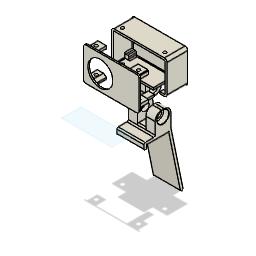
camera_enclosure (Autodesk Fusion 360 design; units mm, degrees)
Autodesk Fusion 360 part; units mm, degrees
sketch "Sketch1" plane through (0, 0, 0) normal (0, 0, 1) x (1, 0, 0)
  line L0 (0, 0) -> (38.5, 0)
  line L1 (38.5, 0) -> (38.5, 21.5)
  line L2 (38.5, 21.5) -> (0, 21.5)
  line L3 (0, 21.5) -> (0, 0)
  dimension "d1" = 38.5
  dimension "d2" = 21.5
  constraint horizontal L0
  constraint vertical L1
  constraint horizontal L2
  constraint vertical L3
  constraint coincident L0.start L3.end
  measures "d1" distance of L0.start L0.end
  measures "d2" distance of L0.start L2.end
extrude "Extrude1" add sketch "Sketch1" along normal blind 2 makes body 1
fillet "Fillet1" radius 2 4 edges at (38.5, 21.5, 1) (0, 21.5, 1) (38.5, 0, 1) (0, 0, 1) on bodies 1
sketch "Sketch2" plane through (0, 0, 2) normal (0, 0, 1) x (1, 0, 0)
  arc A0 (0, 2) -> (2, 0) centre (2, 2) ccw
  line L0 (2, 0) -> (36.5, 0)
  arc A1 (36.5, 0) -> (38.5, 2) centre (36.5, 2) ccw
  line L1 (38.5, 2) -> (38.5, 19.5)
  arc A2 (38.5, 19.5) -> (36.5, 21.5) centre (36.5, 19.5) ccw
  line L2 (36.5, 21.5) -> (2, 21.5)
  arc A3 (2, 21.5) -> (0, 19.5) centre (2, 19.5) ccw
  line L3 (0, 19.5) -> (0, 2)
  circle A4 centre (11, 10) radius 9
  dimension "d7" = 18
  dimension "d8" = 11.5
  dimension "d9" = 11
  measures "d7" diameter of A4
  measures "d8" distance of L2 A4.centre
  measures "d9" distance of L3 A4.centre
extrude "Extrude2" add sketch "Sketch2" along normal blind 20 contours A4 bodies 1
fillet "Fillet2" radius 0.5 1 edges at (2.6091, 6.7455, 22) on bodies 1
sketch "Sketch3" plane through (0, 0, 0) normal (0, 0, -1) x (-1, 0, 0)
  arc A0 (-2, 0) -> (0, 2) centre (-2, 2) ccw
  line L0 (0, 2) -> (0, 19.5)
  arc A1 (0, 19.5) -> (-2, 21.5) centre (-2, 19.5) ccw
  line L1 (-2, 21.5) -> (-36.5, 21.5)
  arc A2 (-36.5, 21.5) -> (-38.5, 19.5) centre (-36.5, 19.5) ccw
  line L2 (-38.5, 19.5) -> (-38.5, 2)
  arc A3 (-38.5, 2) -> (-36.5, 0) centre (-36.5, 2) ccw
  line L3 (-36.5, 0) -> (-2, 0)
  line L4 (-9, 14) -> (-5, 14)
  line L5 (-5, 14) -> (-5, 4)
  line L6 (-5, 4) -> (-9, 4)
  line L7 (-9, 4) -> (-9, 14)
  dimension "d14" = 4
  dimension "d15" = 10
  dimension "d16" = 4
  dimension "d17" = 5
  constraint horizontal L4
  constraint vertical L5
  constraint horizontal L6
  constraint vertical L7
  measures "d14" distance of L5.end L6.end
  measures "d15" distance of L4.start L6.end
  measures "d16" distance of L3 L6
  measures "d17" distance of L0 L5
extrude "Extrude3" add sketch "Sketch3" along normal blind 3 contours L4 L5 L6 L7 bodies 1
fillet "Fillet3" radius 2 2 edges at (9, 9, -3) (5, 9, -3) on bodies 1
sketch "Sketch4" plane through (0, 0, 0) normal (0, 0, -1) x (-1, 0, 0)
  line L0 (-9, 4) -> (-9, 14)
  line L1 (-9, 14) -> (-5, 14)
  line L2 (-5, 14) -> (-5, 4)
  line L3 (-5, 4) -> (-9, 4)
  arc A0 (-2, 0) -> (0, 2) centre (-2, 2) ccw
  line L4 (0, 2) -> (0, 19.5)
  arc A1 (0, 19.5) -> (-2, 21.5) centre (-2, 19.5) ccw
  line L5 (-2, 21.5) -> (-36.5, 21.5)
  arc A2 (-36.5, 21.5) -> (-38.5, 19.5) centre (-36.5, 19.5) ccw
  line L6 (-38.5, 19.5) -> (-38.5, 2)
  arc A3 (-38.5, 2) -> (-36.5, 0) centre (-36.5, 2) ccw
  line L7 (-36.5, 0) -> (-2, 0)
  line L8 (-16, 13) -> (-9, 13)
  line L9 (-9, 13) -> (-9, 6)
  line L10 (-9, 6) -> (-16, 6)
  line L11 (-16, 6) -> (-16, 13)
  dimension "d22" = 7
  dimension "d23" = 7
  dimension "d24" = 6
  constraint horizontal L8
  constraint vertical L9
  constraint horizontal L10
  constraint vertical L11
  constraint collinear L0 L9
  measures "d22" distance of L8.start L8.end
  measures "d23" distance of L8.start L10.end
  measures "d24" distance of L7 L10
extrude "Extrude4" add sketch "Sketch4" along normal blind 1 contours L0 L8 L9 L10 L11 bodies 1
ref_plane "WorkPlane1" through (19.25, 10.75, 10) normal (0, 0, 1) x (1, 0, 0)
sketch "Sketch5" plane through (19.25, 10.75, 10) normal (0, 0, 1) x (1, 0, 0)
  line L0 (19.75, -11.25) -> (-19.75, -11.25)
  line L1 (-19.75, -11.25) -> (-19.75, 11.25)
  line L2 (-19.75, 11.25) -> (19.75, 11.25)
  line L3 (19.75, 11.25) -> (19.75, -11.25)
  line L4 (19.25, -8.75) -> (19.25, 8.75)
  line L5 (-19.25, 8.75) -> (-19.25, -8.75)
  line L6 (17.25, 10.75) -> (-17.25, 10.75)
  line L7 (-17.25, -10.75) -> (17.25, -10.75)
  line L8 (-21.25, -12.75) -> (-21.25, 12.75)
  line L9 (-21.25, 12.75) -> (21.25, 12.75)
  line L10 (21.25, 12.75) -> (21.25, -12.75)
  line L11 (21.25, -12.75) -> (-21.25, -12.75)
  circle A0 centre (-8.25, -0.75) radius 8.5
  circle A1 centre (-8.25, -0.75) radius 9.5
  dimension "d28" = 0.5
  dimension "d29" = 0.5
  dimension "d30" = 0.5
  dimension "d31" = 0.5
  dimension "d32" = -1.5
  dimension "d33" = 19
  constraint horizontal L0
  constraint vertical L1
  constraint horizontal L2
  constraint vertical L3
  constraint concentric A0 A1
  measures "d28" distance of L3 L4
  measures "d29" distance of L1 L5
  measures "d30" distance of L2 L6
  measures "d31" distance of L0 L7
  measures "d33" diameter of A1
extrude "Extrude5" add sketch "Sketch5" along normal blind 1.2 separate body contours L0 L1 L2 L3 | L8 L9 L10 L11 makes body 2
fillet "Fillet4" radius 2 4 edges at (40.5, 23.5, 10.6) (-2, 23.5, 10.6) (-2, -2, 10.6) (40.5, -2, 10.6) on bodies 2
sketch "Sketch6" plane through (0, 0, 10) normal (0, 0, -1) x (-1, 0, 0)
  circle A0 centre (-11, 10) radius 9.5
  arc A1 (-40.5, 0) -> (-38.5, -2) centre (-38.5, 0) ccw
  line L0 (-38.5, -2) -> (0, -2)
  arc A2 (0, -2) -> (2, 0) centre (0, 0) ccw
  line L1 (2, 0) -> (2, 21.5)
  arc A3 (2, 21.5) -> (0, 23.5) centre (0, 21.5) ccw
  line L2 (0, 23.5) -> (-38.5, 23.5)
  arc A4 (-38.5, 23.5) -> (-40.5, 21.5) centre (-38.5, 21.5) ccw
  line L3 (-40.5, 21.5) -> (-40.5, 0)
  line L4 (-39, 21.5) -> (-39, 0)
  arc A5 (-39, 0) -> (-38.5, -0.5) centre (-38.5, 0) ccw
  line L5 (-38.5, -0.5) -> (0, -0.5)
  arc A6 (0, -0.5) -> (0.5, 0) centre (0, 0) ccw
  line L6 (0.5, 0) -> (0.5, 21.5)
  arc A7 (0.5, 21.5) -> (0, 22) centre (0, 21.5) ccw
  line L7 (0, 22) -> (-38.5, 22)
  arc A8 (-38.5, 22) -> (-39, 21.5) centre (-38.5, 21.5) ccw
  dimension "d38" = -1.5
extrude "Extrude6" add sketch "Sketch6" along normal blind 15 separate body contours A1 L0 A2 L1 A3 L2 A4 L3 makes body 3
sketch "Sketch7" plane through (0, 0, -5) normal (0, 0, -1) x (-1, 0, 0)
  arc A0 (-38.5, 22) -> (-39, 21.5) centre (-38.5, 21.5) ccw
  line L0 (-38.5, 22) -> (0, 22)
  arc A1 (0.5, 21.5) -> (0, 22) centre (0, 21.5) ccw
  line L1 (0.5, 21.5) -> (0.5, 0)
  arc A2 (0, -0.5) -> (0.5, 0) centre (0, 0) ccw
  line L2 (0, -0.5) -> (-38.5, -0.5)
  arc A3 (-39, 0) -> (-38.5, -0.5) centre (-38.5, 0) ccw
  line L3 (-39, 0) -> (-39, 21.5)
  line L4 (-40.5, 21.5) -> (-40.5, 0)
  arc A4 (-40.5, 0) -> (-38.5, -2) centre (-38.5, 0) ccw
  line L5 (-38.5, -2) -> (0, -2)
  arc A5 (0, -2) -> (2, 0) centre (0, 0) ccw
  line L6 (2, 0) -> (2, 21.5)
  arc A6 (2, 21.5) -> (0, 23.5) centre (0, 21.5) ccw
  line L7 (0, 23.5) -> (-38.5, 23.5)
  arc A7 (-38.5, 23.5) -> (-40.5, 21.5) centre (-38.5, 21.5) ccw
extrude "Extrude7" add sketch "Sketch7" along normal blind 1.2 contours A0 L0 A1 L1 A2 L2 A3 L3 | L4 A4 L5 A5 L6 A6 L7 A7 bodies 3
sketch "Sketch8" plane through (0, 0, -6.2) normal (0, 0, -1) x (-1, 0, 0)
  arc A0 (-38.5, 23.5) -> (-40.5, 21.5) centre (-38.5, 21.5) ccw
  line L0 (-40.5, 21.5) -> (-40.5, 0)
  arc A1 (-40.5, 0) -> (-38.5, -2) centre (-38.5, 0) ccw
  line L1 (-38.5, -2) -> (0, -2)
  arc A2 (0, -2) -> (2, 0) centre (0, 0) ccw
  line L2 (2, 0) -> (2, 21.5)
  arc A3 (2, 21.5) -> (0, 23.5) centre (0, 21.5) ccw
  line L3 (0, 23.5) -> (-38.5, 23.5)
  circle A4 centre (-32.5, 2.5) radius 2.5
  arc A5 (-38.5, 22) -> (-39, 21.5) centre (-38.5, 21.5) ccw
  line L4 (-39, 21.5) -> (-39, 0)
  arc A6 (-39, 0) -> (-38.5, -0.5) centre (-38.5, 0) ccw
  line L5 (-38.5, -0.5) -> (0, -0.5)
  arc A7 (0, -0.5) -> (0.5, 0) centre (0, 0) ccw
  line L6 (0.5, 0) -> (0.5, 21.5)
  arc A8 (0.5, 21.5) -> (0, 22) centre (0, 21.5) ccw
  line L7 (0, 22) -> (-38.5, 22)
  line L8 (-40.5, 0) -> (-40.5, 21.5)
  arc A9 (-38.5, 23.5) -> (-40.5, 21.5) centre (-38.5, 21.5) ccw
  line L9 (-38.5, 23.5) -> (0, 23.5)
  arc A10 (2, 21.5) -> (0, 23.5) centre (0, 21.5) ccw
  line L10 (2, 21.5) -> (2, 0)
  arc A11 (0, -2) -> (2, 0) centre (0, 0) ccw
  line L11 (0, -2) -> (-38.5, -2)
  arc A12 (-40.5, 0) -> (-38.5, -2) centre (-38.5, 0) ccw
  line L12 (-32.5, 2.5) -> (-30, 2.5) construction
  line L13 (-32.5, 2.5) -> (-35, 2.5) construction
  line L14 (-30, 2.5) -> (-30, -0.5)
  line L15 (-35, 2.5) -> (-35, -0.5)
  dimension "d43" = 5
  dimension "d44" = 4.5
  dimension "d45" = 8
  constraint coincident A4.centre L12.start
  constraint coincident A4 L12.end
  constraint horizontal L12
  constraint coincident A4 L13.end
  constraint parallel L12 L13
  constraint coincident L5 L14.end
  constraint tangent A4 L14
  constraint coincident L5 L15.end
  constraint tangent A4 L15
  measures "d43" diameter of A4
  measures "d44" distance of L1 A4.centre
  measures "d45" distance of L0 A4.centre
extrude "Extrude22" cut sketch "Sketch8" against normal blind 1.2 contours A4 L5 L14 L15 bodies 3
extrude "Extrude8" cut sketch "Sketch8" against normal blind 1.2 contours A4 bodies 3
sketch "Sketch21" plane through (0, -0.5, 0) normal (0, 1, 0) x (-1, 0, 0)
  line L0 (0, 10) -> (-38.5, 10)
  line L1 (-38.5, 10) -> (-38.5, -5)
  line L2 (-38.5, -5) -> (-35, -5)
  line L3 (-35, -5) -> (-35, -6.2)
  line L4 (-35, -6.2) -> (-30, -6.2)
  line L5 (-30, -6.2) -> (-30, -5)
  line L6 (-30, -5) -> (0, -5)
  line L7 (0, -5) -> (0, 10)
sketch "Sketch22" plane through (0, -2, 0) normal (0, -1, 0) x (1, 0, 0)
  line L0 (38.5, 10) -> (0, 10)
  line L1 (0, 10) -> (0, -6.2)
  line L2 (0, -6.2) -> (38.5, -6.2)
  line L3 (38.5, -6.2) -> (38.5, 10)
  line L4 (30, -6.2) -> (30, -5)
  line L5 (30, -5) -> (30, -6.2)
  line L6 (35, -6.2) -> (35, -5)
  line L7 (35, -5) -> (35, -6.2)
  line L8 (35, -6.2) -> (30, -6.2)
  line L9 (30, -5) -> (30, 10)
  line L10 (35, -5) -> (35, 10)
  line L11 (30, 10) -> (35, 10)
  constraint coincident L6.start L7.end
  constraint coincident L4.start L5.end
  constraint coincident L4.end L5.start
  constraint coincident L0 L9.end
  constraint perpendicular L0 L9
  constraint coincident L6.end L7.start
  constraint coincident L0 L10.end
  constraint perpendicular L0 L10
extrude "Extrude23" cut sketch "Sketch22" against normal blind 1.5 contours L0 L2 L4 L5 L6 L7 L8 L9 L10 L11 bodies 3
chamfer "Chamfer1" distance 0.5 angle 45 8 edges at (19.25, 22, -5) (-0.3536, 21.8536, -5) (-0.5, 10.75, -5) (-0.3536, -0.3536, -5) (19.25, -0.5, -5) (38.8536, -0.3536, -5) (39, 10.75, -5) (38.8536, 21.8536, -5) on bodies 3
fillet "Fillet5" radius 0.3 8 edges at (40.5, 10.75, -6.2) (39.9142, -1.4142, -6.2) (19.25, -2, -6.2) (-1.4142, -1.4142, -6.2) (-2, 10.75, -6.2) (-1.4142, 22.9142, -6.2) (19.25, 23.5, -6.2) (39.9142, 22.9142, -6.2) on bodies 3
sketch "Sketch10" plane through (0, 0, 22) normal (0, 0, 1) x (1, 0, 0)
  circle A0 centre (11, 10) radius 8.5
  circle A1 centre (11, 10) radius 6.0027
  constraint concentric A0 A1
extrude "Extrude10" cut sketch "Sketch10" against normal blind 5 contours A1 bodies 1
chamfer "Chamfer3" distance 2 angle 45 2 edges at (5.4035, 12.1707, 22) (5.4035, 12.1707, 17) on bodies 1
move_body "Move1" bodies 3 to x (1, 0, 0) y (0, 1, 0) z (0, 0, 1) at (0, 0, -40)
move_body "Move2" bodies 1 to x (1, 0, 0) y (0, 1, 0) z (0, 0, 1) at (0, 0, -20)
ref_plane "WorkPlane2" through (19.25, 10.75, -37.95) normal (1, 0, 0) x (0, -1, 0)
sketch "Sketch11" plane through (19.25, 10.75, -37.95) normal (1, 0, 0) x (0, 0, -1)
  line L0 (7.95, -12.75) -> (7.95, -10.75)
  line L1 (7.95, -10.75) -> (-7.95, -10.75)
  line L2 (-7.95, -12.75) -> (-7.95, -10.75)
  line L3 (-7.95, -12.75) -> (7.95, -12.75)
  line L4 (-5.85, -12.75) -> (6.15, -12.75)
  line L5 (6.15, -12.75) -> (6.15, -24.75)
  line L6 (6.15, -24.75) -> (-5.85, -24.75)
  line L7 (-5.85, -24.75) -> (-5.85, -12.75)
  line L8 (8.25, -10.75) -> (8.25, 10.75)
  dimension "d71" = 2.1
  dimension "d73" = 12
  dimension "d74" = 2.2
  dimension "d75" = 12
  constraint horizontal L4
  constraint vertical L5
  constraint horizontal L6
  constraint vertical L7
  constraint coincident L3 L4.start
  measures "d71" distance of L5 L8
  measures "d73" distance of L5 L7
  measures "d75" distance of L4.start L6.end
extrude "Extrude11" add sketch "Sketch11" along normal mid plane 6 contours L3 L4 L5 L6 L7 bodies 3
ref_plane "WorkPlane3" through (22.55, -8, -38.1) normal (1, 0, 0) x (0, 0, -1)
sketch "Sketch12" plane through (22.55, -8, -38.1) normal (1, 0, 0) x (0, 0, -1)
  line L0 (-6, -6) -> (6, -6)
  line L1 (6, -6) -> (6, 6)
  line L2 (6, 6) -> (-6, 6)
  line L3 (-6, 6) -> (-6, -6)
  line L4 (6, 4) -> (-6, 4)
  line L5 (-6, -6) -> (6, -6)
  line L6 (6, -6) -> (6, -11)
  line L7 (6, -11) -> (-6, -11)
  line L8 (-6, -11) -> (-6, -6)
  dimension "d79" = 2
  dimension "d80" = 5
  constraint coincident L1 L4.start
  constraint coincident L3 L4.end
  constraint perpendicular L3 L4
  constraint horizontal L5
  constraint vertical L6
  constraint horizontal L7
  constraint vertical L8
  constraint coincident L0.start L3.end
  constraint collinear L1 L6
  measures "d79" distance of L2 L4
  measures "d80" distance of L0.end L6.end
extrude "Extrude12" add sketch "Sketch12" along normal blind 3 separate body contours L0 L1 L3 L4 L5 | L0 L5 L6 L7 L8 makes body 4
ref_plane "WorkPlane4" through (19.25, -8, -38.1) normal (-1, 0, 0) x (0, 0, 1)
mirror "Mirror1" about plane through (19.25, -8, -38.1) normal (-1, 0, 0) of bodies 4 makes body 5
sketch "Sketch13" plane through (0, -19, 0) normal (0, -1, 0) x (1, 0, 0)
  line L0 (22.55, -32.1) -> (22.55, -44.1)
  line L1 (22.55, -44.1) -> (25.55, -44.1)
  line L2 (25.55, -44.1) -> (25.55, -32.1)
  line L3 (25.55, -32.1) -> (22.55, -32.1)
  line L4 (15.95, -44.1) -> (15.95, -32.1)
  line L5 (15.95, -32.1) -> (12.95, -32.1)
  line L6 (12.95, -32.1) -> (12.95, -44.1)
  line L7 (12.95, -44.1) -> (15.95, -44.1)
  line L8 (15.95, -32.1) -> (22.55, -32.1)
  line L9 (22.55, -32.1) -> (22.55, -44.1)
  line L10 (22.55, -44.1) -> (15.95, -44.1)
  line L11 (15.95, -44.1) -> (15.95, -32.1)
  constraint horizontal L8
  constraint vertical L9
  constraint horizontal L10
  constraint vertical L11
  constraint coincident L0.end L1.start
  constraint coincident L4.end L5.start
extrude "Extrude13" add sketch "Sketch13" against normal blind 2 contours L0 L4 L8 L9 L10 L11 bodies 4 5
fillet "Fillet7" radius 5 6 edges at (19.25, -14, -32.1) (19.25, -14, -44.1) (24.05, -4, -44.1) (24.05, -4, -32.1) (14.45, -4, -32.1) (14.45, -4, -44.1) on bodies 3 4
sketch "Sketch14" plane through (12.95, 0, 0) normal (-1, 0, 0) x (0, 0, 1)
  arc A0 (-39.1, -4) -> (-44.1, -9) centre (-39.1, -9) ccw
  line L0 (-44.1, -9) -> (-44.1, -19)
  line L1 (-44.1, -19) -> (-32.1, -19)
  line L2 (-32.1, -19) -> (-32.1, -9)
  arc A1 (-32.1, -9) -> (-37.1, -4) centre (-37.1, -9) ccw
  line L3 (-37.1, -4) -> (-39.1, -4)
  circle A2 centre (-38.1, -9) radius 3
  dimension "d90" = 6
  dimension "d91" = 6
  dimension "d92" = 6
  dimension "d93" = 5
  measures "d90" distance of L2 A2.centre
  measures "d91" distance of L0 A2.centre
  measures "d92" diameter of A2
  measures "d93" distance of L3 A2.centre
extrude "Extrude14" cut sketch "Sketch14" against normal blind 13 contours A2 bodies 3 4
sketch "Sketch15" plane through (12.95, 0, 0) normal (-1, 0, 0) x (0, 0, 1)
  circle A0 centre (-38.1, -9) radius 3
  arc A1 (-39.1, -4) -> (-44.1, -9) centre (-39.1, -9) ccw
  line L0 (-44.1, -9) -> (-44.1, -19)
  line L1 (-44.1, -19) -> (-32.1, -19)
  line L2 (-32.1, -19) -> (-32.1, -9)
  arc A2 (-32.1, -9) -> (-37.1, -4) centre (-37.1, -9) ccw
  line L3 (-37.1, -4) -> (-39.1, -4)
  line L4 (-35.6751, -4.8) -> (-40.5249, -4.8)
  line L5 (-40.5249, -4.8) -> (-42.9497, -9)
  line L6 (-42.9497, -9) -> (-40.5249, -13.2)
  line L7 (-40.5249, -13.2) -> (-35.6751, -13.2)
  line L8 (-35.6751, -13.2) -> (-33.2503, -9)
  line L9 (-33.2503, -9) -> (-35.6751, -4.8)
  line L10 (-42.9497, -9) -> (-33.2503, -9) construction
  point P0 (-38.1, -9)
  dimension "d96" = 4.2
  constraint coincident P0 A0.centre
  constraint parallel L1 L7
  measures "d96" distance of P0 L9
extrude "Extrude15" add sketch "Sketch15" along normal blind 4 contours A1 L0 L1 L2 A2 L3 bodies 4
sketch "Sketch16" plane through (25.55, 0, 0) normal (1, 0, 0) x (0, 0, -1)
  circle A0 centre (38.1, -9) radius 3
  arc A1 (37.1, -4) -> (32.1, -9) centre (37.1, -9) ccw
  line L0 (32.1, -9) -> (32.1, -19)
  line L1 (32.1, -19) -> (44.1, -19)
  line L2 (44.1, -19) -> (44.1, -9)
  arc A2 (44.1, -9) -> (39.1, -4) centre (39.1, -9) ccw
  line L3 (39.1, -4) -> (37.1, -4)
  circle A3 centre (38.1, -9) radius 4.5
  dimension "d99" = 9
  constraint concentric A0 A3
  measures "d99" diameter of A3
extrude "Extrude16" add sketch "Sketch16" along normal blind 4 contours A1 L0 L1 L2 A2 L3 bodies 4
chamfer "Chamfer4" distance 0.2 angle 45 6 edges at (8.95, -4.8, -38.1) (8.95, -6.9, -41.7373) (8.95, -11.1, -41.7373) (8.95, -6.9, -34.4627) (8.95, -11.1, -34.4627) (8.95, -13.2, -38.1) on bodies 4
chamfer "Chamfer5" distance 0.2 angle 45 1 edges at (29.55, -7.3727, -33.9045) on bodies 4
move_body "Move3" bodies 3 1 2 to x (1, 0, 0) y (0, 1, 0) z (0, 0, 1) at (0, 15, 0)
sketch "Sketch17" plane through (29.55, 0, 0) normal (1, 0, 0) x (0, 0, -1)
  line L0 (39.1, -4) -> (37.1, -4)
  arc A0 (37.1, -4) -> (32.1, -9) centre (37.1, -9) ccw
  line L1 (32.1, -9) -> (32.1, -19)
  line L2 (32.1, -19) -> (44.1, -19)
  line L3 (44.1, -19) -> (44.1, -9)
  arc A1 (44.1, -9) -> (39.1, -4) centre (39.1, -9) ccw
  circle A2 centre (38.1, -9) radius 4.7
  line L4 (32.1, -19) -> (23.4688, -19)
  line L5 (23.4688, -19) -> (23.4688, -24)
  line L6 (23.4688, -24) -> (25.4688, -24)
  line L7 (25.4688, -24) -> (25.4688, -21)
  line L8 (25.4688, -21) -> (42.4688, -21)
  line L9 (42.4688, -21) -> (51.5173, -65.0809)
  line L10 (51.5173, -65.0809) -> (53.4765, -64.6787)
  line L11 (53.4765, -64.6787) -> (44.1, -19)
  dimension "d104" = 2
  dimension "d105" = 17
  dimension "d107" = 2
  dimension "d108" = 2
  dimension "d109" = 45
  dimension "d110" = 11.6
  dimension "d111" = 5
  constraint coincident L1.end L2.start
  constraint perpendicular L1 L4
  constraint perpendicular L4 L5
  constraint perpendicular L5 L6
  constraint perpendicular L6 L7
  constraint perpendicular L7 L8
  constraint perpendicular L9 L10
  constraint perpendicular L10 L11
  constraint coincident L2.end L3.start
  measures "d104" distance of L9 L11
  measures "d105" distance of L7 L8.end
  measures "d107" distance of L5 L7
  measures "d108" distance of L2 L8
  measures "d109" distance of L8.end L9.end
  measures "d110" angle of L7 L9
  measures "d111" distance of L4 L6
extrude "Extrude18" add sketch "Sketch17" against normal blind 20.6 contours L2 L4 L5 L6 L7 L8 L9 L10 L11 bodies 4
extrude "Extrude17" add sketch "Sketch17" against normal blind 20.6 contours L2 L4 L5 L6 L7 L8 L9 L10 L11 bodies 4
fillet "Fillet8" radius 10 1 edges at (19.25, -19, -44.1) on bodies 4
sketch "Sketch18" plane through (8.95, 0, 0) normal (-1, 0, 0) x (0, 0, 1)
  line L0 (-35.5597, -13.4) -> (-40.6403, -13.4)
  line L1 (-40.6403, -13.4) -> (-43.1807, -9)
  line L2 (-43.1807, -9) -> (-40.6403, -4.6)
  line L3 (-40.6403, -4.6) -> (-35.5597, -4.6)
  line L4 (-35.5597, -4.6) -> (-33.0193, -9)
  line L5 (-33.0193, -9) -> (-35.5597, -13.4)
  line L6 (-32.1, -19) -> (-32.1, -9)
  arc A0 (-32.1, -9) -> (-37.1, -4) centre (-37.1, -9) ccw
  line L7 (-37.1, -4) -> (-39.1, -4)
  arc A1 (-39.1, -4) -> (-44.1, -9) centre (-39.1, -9) ccw
  line L8 (-44.1, -9) -> (-44.1, -17.9842)
  arc A2 (-44.3042, -19.995) -> (-44.1, -17.9842) centre (-54.1, -17.9842) ccw
  line L9 (-44.3042, -19.995) -> (-53.4765, -64.6787)
  line L10 (-53.4765, -64.6787) -> (-51.5173, -65.0809)
  line L11 (-51.5173, -65.0809) -> (-42.4688, -21)
  line L12 (-42.4688, -21) -> (-25.4688, -21)
  line L13 (-25.4688, -21) -> (-25.4688, -24)
  line L14 (-25.4688, -24) -> (-23.4688, -24)
  line L15 (-23.4688, -24) -> (-23.4688, -19)
  line L16 (-23.4688, -19) -> (-32.1, -19)
  circle A3 centre (-42.4688, -21) radius 0.4
  circle A4 centre (-25.4688, -21) radius 0.4
  dimension "d118" = 0.8
  dimension "d119" = 0.8
  constraint coincident L11.end L12.start
  constraint coincident L12.end L13.start
  measures "d118" diameter of A3
  measures "d119" diameter of A4
extrude "Extrude19" cut sketch "Sketch18" against normal blind 20.6 contours L12 L13 A4 | L11 L12 A3 picked at (-25.4688, -20.7341) picked at (-42.693, -21.1431) bodies 4
fillet "Fillet9" radius 1 8 edges at (19.25, -24, -25.4688) (19.25, -24, -23.4688) (19.25, -19, -23.4688) (19.25, -19, -32.1) (19.25, -65.0809, -51.5173) (19.25, -64.6787, -53.4765) (19.25, -17, -44.1) (19.25, -17, -32.1) on bodies 4
sketch "Sketch20" plane through (0, 0, -45) normal (0, 0, 1) x (1, 0, 0)
  line L0 (38.5, 36.5) -> (0, 36.5)
  line L1 (0, 36.5) -> (0, 15)
  line L2 (35, 15) -> (38.5, 15)
  line L3 (38.5, 15) -> (38.5, 36.5)
  arc A0 (39, 36.5) -> (38.5, 37) centre (38.5, 36.5) ccw
  line L4 (39, 36.5) -> (39, 15)
  arc A1 (38.5, 14.5) -> (39, 15) centre (38.5, 15) ccw
  line L5 (30, 14.5) -> (0, 14.5)
  arc A2 (-0.5, 15) -> (0, 14.5) centre (0, 15) ccw
  line L6 (-0.5, 15) -> (-0.5, 36.5)
  arc A3 (0, 37) -> (-0.5, 36.5) centre (0, 36.5) ccw
  line L7 (0, 37) -> (38.5, 37)
  line L8 (40.5, 15) -> (40.5, 36.5)
  arc A4 (40.5, 36.5) -> (38.5, 38.5) centre (38.5, 36.5) ccw
  line L9 (38.5, 38.5) -> (0, 38.5)
  arc A5 (0, 38.5) -> (-2, 36.5) centre (0, 36.5) ccw
  line L10 (-2, 36.5) -> (-2, 15)
  arc A6 (-2, 15) -> (0, 13) centre (0, 15) ccw
  line L11 (35, 13) -> (38.5, 13)
  arc A7 (38.5, 13) -> (40.5, 15) centre (38.5, 15) ccw
  line L12 (2.5, 37) -> (2.5, 34)
  line L13 (2.5, 34) -> (-0.5, 34)
  line L14 (36, 37) -> (36, 34)
  line L15 (36, 34) -> (39, 34)
  line L16 (36, 14.5) -> (36, 17.5)
  line L17 (36, 17.5) -> (39, 17.5)
  line L18 (-0.5, 17.5) -> (2.5, 17.5)
  line L19 (2.5, 17.5) -> (2.5, 14.5)
  line L20 (0, 15) -> (30, 15)
  line L21 (30, 15) -> (30, 17.5)
  arc A8 (35, 17.5) -> (30, 17.5) centre (32.5, 17.5) ccw
  line L22 (35, 17.5) -> (35, 15)
  line L23 (30, 13) -> (30, 14.5)
  line L24 (38.5, 14.5) -> (35, 14.5)
  line L25 (35, 14.5) -> (35, 13)
  line L26 (0, 13) -> (30, 13)
  dimension "d130" = 3
  dimension "d131" = 3
  dimension "d132" = 3
  dimension "d133" = 3
  dimension "d134" = 3
  dimension "d135" = 3
  dimension "d136" = 3
  dimension "d137" = 3
  constraint coincident L7 L12.start
  constraint perpendicular L0 L12
  constraint coincident L6 L13.end
  constraint perpendicular L6 L13
  constraint coincident L7 L14.start
  constraint perpendicular L0 L14
  constraint coincident L4 L15.end
  constraint perpendicular L4 L15
  constraint coincident L5 L16.start
  constraint perpendicular L2 L16
  constraint coincident L4 L17.end
  constraint perpendicular L4 L17
  constraint coincident L6 L18.start
  constraint perpendicular L1 L18
  constraint coincident L5 L19.end
  constraint perpendicular L5 L19
  measures "d130" distance of L12.start L12.end
  measures "d131" distance of L12.end L13.end
  measures "d132" distance of L18.end L19.end
  measures "d133" distance of L18.start L18.end
  measures "d134" distance of L14.start L14.end
  measures "d135" distance of L14.end L15.end
  measures "d136" distance of L16.end L17.end
  measures "d137" distance of L16.start L16.end
extrude "Extrude21" add sketch "Sketch20" along normal blind 6 contours L0 L3 L14 L15 | L0 L3 A0 L4 L7 L14 L15 | L0 L1 L12 L13 | L0 L1 L6 A3 L7 L12 L13 | L2 L3 L4 A1 L16 L17 L24 | L2 L3 L16 L17 | L1 L18 L19 L20 | L1 L5 A2 L6 L18 L19 L20 bodies 3
fillet "Fillet10" radius 0.8 12 edges at (39, 34, -41.75) (36, 37, -41.75) (36, 34, -42) (39, 17.5, -41.75) (36, 17.5, -42) (36, 14.5, -41.75) (2.5, 37, -41.75) (2.5, 34, -42) (-0.5, 34, -41.75) (-0.5, 17.5, -41.75) (2.5, 17.5, -42) (2.5, 14.5, -41.75) on bodies 3
move_body "Move4" bodies 2 to x (1, 0, 0) y (0, 1, 0) z (0, 0, 1) at (0, 0, -40)
sketch "Sketch23" plane through (0, 0, -30) normal (0, 0, -1) x (-1, 0, 0)
  circle A0 centre (-11, 25) radius 9.5
  arc A1 (-40.5, 15) -> (-38.5, 13) centre (-38.5, 15) ccw
  line L0 (-38.5, 13) -> (0, 13)
  arc A2 (0, 13) -> (2, 15) centre (0, 15) ccw
  line L1 (2, 15) -> (2, 36.5)
  arc A3 (2, 36.5) -> (0, 38.5) centre (0, 36.5) ccw
  line L2 (0, 38.5) -> (-38.5, 38.5)
  arc A4 (-38.5, 38.5) -> (-40.5, 36.5) centre (-38.5, 36.5) ccw
  line L3 (-40.5, 36.5) -> (-40.5, 15)
  arc A5 (-2.5, 34.8) -> (-1.7, 34) centre (-1.7, 34.8) ccw
  line L4 (-2.5, 34.8) -> (-2.5, 36.2)
  arc A6 (-2.5, 36.2) -> (-3.3, 37) centre (-3.3, 36.2) ccw
  line L5 (-3.3, 37) -> (0, 37)
  arc A7 (0.5, 36.5) -> (0, 37) centre (0, 36.5) ccw
  line L6 (0.5, 36.5) -> (0.5, 33.2)
  arc A8 (0.5, 33.2) -> (-0.3, 34) centre (-0.3, 33.2) ccw
  line L7 (-0.3, 34) -> (-1.7, 34)
  arc A9 (-1.7, 17.5) -> (-2.5, 16.7) centre (-1.7, 16.7) ccw
  line L8 (-1.7, 17.5) -> (-0.3, 17.5)
  arc A10 (-0.3, 17.5) -> (0.5, 18.3) centre (-0.3, 18.3) ccw
  line L9 (0.5, 18.3) -> (0.5, 15)
  arc A11 (0, 14.5) -> (0.5, 15) centre (0, 15) ccw
  line L10 (0, 14.5) -> (-3.3, 14.5)
  arc A12 (-3.3, 14.5) -> (-2.5, 15.3) centre (-3.3, 15.3) ccw
  line L11 (-2.5, 15.3) -> (-2.5, 16.7)
  arc A13 (-36, 16.7) -> (-36.8, 17.5) centre (-36.8, 16.7) ccw
  line L12 (-36, 16.7) -> (-36, 15.3)
  arc A14 (-36, 15.3) -> (-35.2, 14.5) centre (-35.2, 15.3) ccw
  line L13 (-35.2, 14.5) -> (-38.5, 14.5)
  arc A15 (-39, 15) -> (-38.5, 14.5) centre (-38.5, 15) ccw
  line L14 (-39, 15) -> (-39, 18.3)
  arc A16 (-39, 18.3) -> (-38.2, 17.5) centre (-38.2, 18.3) ccw
  line L15 (-38.2, 17.5) -> (-36.8, 17.5)
  arc A17 (-36.8, 34) -> (-36, 34.8) centre (-36.8, 34.8) ccw
  line L16 (-36.8, 34) -> (-38.2, 34)
  arc A18 (-38.2, 34) -> (-39, 33.2) centre (-38.2, 33.2) ccw
  line L17 (-39, 33.2) -> (-39, 36.5)
  arc A19 (-38.5, 37) -> (-39, 36.5) centre (-38.5, 36.5) ccw
  line L18 (-38.5, 37) -> (-35.2, 37)
  arc A20 (-35.2, 37) -> (-36, 36.2) centre (-35.2, 36.2) ccw
  line L19 (-36, 36.2) -> (-36, 34.8)
extrude "Extrude24" add sketch "Sketch23" along normal up to surface (7.8 mm away) contours A5 L4 A6 L5 A7 L6 A8 L7 | A9 L8 A10 L9 A11 L10 A12 L11 | A13 L12 A14 L13 A15 L14 A16 L15 | A17 L16 A18 L17 A19 L18 A20 L19 bodies 2
sketch "Sketch24" plane through (0, 0, -37.8) normal (0, 0, -1) x (-1, 0, 0)
  line L0 (-35.2, 37) -> (-38.5, 37)
  arc A0 (-38.5, 37) -> (-39, 36.5) centre (-38.5, 36.5) ccw
  line L1 (-39, 36.5) -> (-39, 33.2)
  arc A1 (-38.2, 34) -> (-39, 33.2) centre (-38.2, 33.2) ccw
  line L2 (-38.2, 34) -> (-36.8, 34)
  arc A2 (-36.8, 34) -> (-36, 34.8) centre (-36.8, 34.8) ccw
  line L3 (-36, 34.8) -> (-36, 36.2)
  arc A3 (-35.2, 37) -> (-36, 36.2) centre (-35.2, 36.2) ccw
  line L4 (-38.2, 34) -> (-39, 34)
  line L5 (-36, 36.2) -> (-36, 37)
  line L6 (0.5, 33.2) -> (0.5, 36.5)
  arc A4 (0.5, 36.5) -> (0, 37) centre (0, 36.5) ccw
  line L7 (0, 37) -> (-3.3, 37)
  arc A5 (-2.5, 36.2) -> (-3.3, 37) centre (-3.3, 36.2) ccw
  line L8 (-2.5, 36.2) -> (-2.5, 34.8)
  arc A6 (-2.5, 34.8) -> (-1.7, 34) centre (-1.7, 34.8) ccw
  line L9 (-1.7, 34) -> (-0.3, 34)
  arc A7 (0.5, 33.2) -> (-0.3, 34) centre (-0.3, 33.2) ccw
  line L10 (-3.3, 14.5) -> (0, 14.5)
  arc A8 (0, 14.5) -> (0.5, 15) centre (0, 15) ccw
  line L11 (0.5, 15) -> (0.5, 18.3)
  arc A9 (-0.3, 17.5) -> (0.5, 18.3) centre (-0.3, 18.3) ccw
  line L12 (-0.3, 17.5) -> (-1.7, 17.5)
  arc A10 (-1.7, 17.5) -> (-2.5, 16.7) centre (-1.7, 16.7) ccw
  line L13 (-2.5, 16.7) -> (-2.5, 15.3)
  arc A11 (-3.3, 14.5) -> (-2.5, 15.3) centre (-3.3, 15.3) ccw
  line L14 (-39, 18.3) -> (-39, 15)
  arc A12 (-39, 15) -> (-38.5, 14.5) centre (-38.5, 15) ccw
  line L15 (-38.5, 14.5) -> (-35.2, 14.5)
  arc A13 (-36, 15.3) -> (-35.2, 14.5) centre (-35.2, 15.3) ccw
  line L16 (-36, 15.3) -> (-36, 16.7)
  arc A14 (-36, 16.7) -> (-36.8, 17.5) centre (-36.8, 16.7) ccw
  line L17 (-36.8, 17.5) -> (-38.2, 17.5)
  arc A15 (-39, 18.3) -> (-38.2, 17.5) centre (-38.2, 18.3) ccw
  line L18 (-0.3, 34) -> (0.5, 34)
  line L19 (-2.5, 36.2) -> (-2.5, 37)
  line L20 (-0.3, 17.5) -> (0.5, 17.5)
  line L21 (-2.5, 15.3) -> (-2.5, 14.5)
  line L22 (-36, 15.3) -> (-36, 14.5)
  line L23 (-38.2, 17.5) -> (-39, 17.5)
  line L24 (-38.8, 34) -> (-38.8, 36.9)
  line L25 (-36, 36.8) -> (-38.9, 36.8)
  line L26 (-2.5, 36.8) -> (0.4, 36.8)
  line L27 (0.3, 34) -> (0.3, 36.9)
  line L28 (0.3, 17.5) -> (0.3, 14.6)
  line L29 (-2.5, 14.7) -> (0.4, 14.7)
  line L30 (-36, 14.7) -> (-38.9, 14.7)
  line L31 (-38.8, 17.5) -> (-38.8, 14.6)
  dimension "d149" = 0.2
  dimension "d150" = 0.2
  dimension "d151" = 0.2
  dimension "d152" = 0.2
  dimension "d153" = 0.2
  dimension "d154" = 0.2
  dimension "d155" = 0.2
  dimension "d156" = 0.2
  constraint coincident A1.start L2.start
  constraint coincident L1 L4.end
  constraint tangent A1 L4
  constraint coincident L3.end A3.end
  constraint coincident L0 L5.end
  constraint tangent A3 L5
  constraint coincident L9.end A7.end
  constraint coincident L6 L18.end
  constraint tangent A7 L18
  constraint coincident A5.start L8.start
  constraint coincident L7 L19.end
  constraint tangent A5 L19
  constraint coincident A9.start L12.start
  constraint coincident L11 L20.end
  constraint tangent A9 L20
  constraint coincident L13.end A11.end
  constraint coincident L10 L21.end
  constraint tangent A11 L21
  constraint coincident A13.start L16.start
  constraint coincident L15 L22.end
  constraint tangent A13 L22
  constraint coincident L17.end A15.end
  constraint coincident L14 L23.end
  constraint tangent A15 L23
  constraint coincident L4 L24.start
  constraint perpendicular L0 L24
  constraint coincident A0 L24.end
  constraint coincident L5 L25.start
  constraint coincident A0 L25.end
  constraint perpendicular L24 L25
  constraint coincident L19 L26.start
  constraint coincident A4 L26.end
  constraint perpendicular L19 L26
  constraint coincident L18 L27.start
  constraint coincident A4 L27.end
  constraint perpendicular L26 L27
  constraint coincident L20 L28.start
  constraint coincident A8 L28.end
  constraint perpendicular L20 L28
  constraint coincident L21 L29.start
  constraint coincident A8 L29.end
  constraint perpendicular L21 L29
  constraint coincident L22 L30.start
  constraint coincident A12 L30.end
  constraint perpendicular L22 L30
  constraint coincident L23 L31.start
  constraint coincident A12 L31.end
  constraint perpendicular L30 L31
  measures "d149" distance of L1 L24
  measures "d150" distance of L0 L25
  measures "d151" distance of L6 L27
  measures "d152" distance of L7 L26
  measures "d153" distance of L10 L29
  measures "d154" distance of L11 L28
  measures "d155" distance of L14 L31
  measures "d156" distance of L15 L30
extrude "Extrude25" cut sketch "Sketch24" against normal blind 7.8 contours L0 A3 L5 | L0 A0 L5 L24 L25 | A0 L24 L25 | A0 L1 L4 L24 L25 | L1 A1 L4 | L6 A7 L18 | L6 A4 L18 L26 L27 | A4 L26 L27 | A4 L7 L19 L26 L27 | L7 A5 L19 | L10 A11 L21 | L10 A8 L21 L28 L29 | A8 L28 L29 | A8 L11 L20 L28 L29 | L11 A9 L20 | L14 A15 L23 | L14 A12 L23 L30 L31 | A12 L30 L31 | A12 L15 L22 L30 L31 | L15 A13 L22 bodies 2
fillet "Fillet11" radius 1 12 edges at (0.7, 34, -30) (2.2657, 34.2343, -30) (2.5, 35.8, -30) (37.8, 34, -30) (36.2343, 34.2343, -30) (36, 35.8, -30) (37.8, 17.5, -30) (36.2343, 17.2657, -30) (36, 15.7, -30) (2.5, 15.7, -30) (2.2657, 17.2657, -30) (0.7, 17.5, -30) on bodies 2
move_body "Move5" bodies 2 to x (1, 0, 0) y (0, 1, 0) z (0, 0, 1) at (0, 0, 20)
extrude "Extrude26" add 2 faces at (38.8, 15.6333, -12.9333) (38.8, 35.8667, -12.9333) along direction (-1, 0, 0) blind 8 on bodies 2 bodies 2
fillet "Fillet12" radius 0.8 4 edges at (30.8, 34, -14.4) (30.8, 33.7071, -10.2929) (30.8, 17.7929, -10.2929) (30.8, 17.5, -14.4) on bodies 2
sketch "Sketch25" plane through (0, 36.8, 0) normal (0, 1, 0) x (-1, 0, 0)
  line L0 (-38.8, -17.8) -> (-30.8, -17.8)
  line L1 (-30.8, -17.8) -> (-30.8, -10)
  line L2 (-30.8, -10) -> (-38.8, -10)
  line L3 (-38.8, -10) -> (-38.8, -17.8)
  circle A0 centre (-35, -14) radius 1.25
  dimension "d165" = 4
  dimension "d166" = 3.8
  dimension "d167" = 2.5
  measures "d165" distance of L2 A0.centre
  measures "d166" distance of L3 A0.centre
  measures "d167" diameter of A0
extrude "Extrude27" cut sketch "Sketch25" against normal blind 22.1 contours A0 bodies 2
extrude "Extrude28" add 2 faces at (-0.3, 35.8667, -12.9333) (-0.3, 15.6333, -12.9333) along direction (1, 0, 0) blind 7 on bodies 2 bodies 2
sketch "Sketch26" plane through (0, 0, -8.8) normal (0, 0, 1) x (1, 0, 0)
  arc A0 (38.5, 13) -> (40.5, 15) centre (38.5, 15) ccw
  line L0 (40.5, 15) -> (40.5, 36.5)
  arc A1 (40.5, 36.5) -> (38.5, 38.5) centre (38.5, 36.5) ccw
  line L1 (38.5, 38.5) -> (0, 38.5)
  arc A2 (0, 38.5) -> (-2, 36.5) centre (0, 36.5) ccw
  line L2 (-2, 36.5) -> (-2, 15)
  arc A3 (-2, 15) -> (0, 13) centre (0, 15) ccw
  line L3 (0, 13) -> (38.5, 13)
  circle A4 centre (11, 25) radius 9.5
  circle A5 centre (11, 25) radius 9.5
extrude "Extrude29" cut sketch "Sketch26" against normal blind 9 contours A4 A5 bodies 2
sketch "Sketch27" plane through (0, 0, -17.8) normal (0, 0, -1) x (-1, 0, 0)
  line L0 (0.3, 36.8) -> (-6.7, 36.8)
  line L1 (-6.7, 36.8) -> (-6.7, 34)
  line L2 (-6.7, 34) -> (0.3, 34)
  line L3 (0.3, 34) -> (0.3, 36.8)
fillet "Fillet13" radius 1 2 edges at (6.7, 33.8577, -10.4858) (6.7, 34, -14.4) on bodies 2
sketch "Sketch28" plane through (0, 0, -10) normal (0, 0, -1) x (-1, 0, 0)
  arc A0 (-4.0718, 18.5) -> (-6.7, 16.5289) centre (-11, 25) ccw
  line L0 (-4.0718, 18.5) -> (0.3, 18.5)
  line L1 (0.3, 18.5) -> (0.3, 14.7)
  line L2 (0.3, 14.7) -> (-6.7, 14.7)
  line L3 (-6.7, 14.7) -> (-6.7, 16.5289)
  line L4 (-30.8, 14.7) -> (-38.8, 14.7)
  line L5 (-38.8, 14.7) -> (-38.8, 18.5)
  line L6 (-38.8, 18.5) -> (-31.6, 18.5)
  spline S0 degree 3 poles (-31.6, 18.5) (-31.3774, 18.2511) (-31.1144, 17.9487) (-30.8711, 17.4599) (-30.8, 17.2155) (-30.8, 17.0033) knots 0 0 0 0 0.100179 0.100179 0.163817 0.163817 0.163817 0.163817
  line L7 (-30.8, 17.0033) -> (-30.8, 14.7)
  arc A1 (-40.5, 15) -> (-38.5, 13) centre (-38.5, 15) ccw
  line L8 (-38.5, 13) -> (0, 13)
  arc A2 (0, 13) -> (2, 15) centre (0, 15) ccw
  line L9 (2, 15) -> (2, 36.5)
  arc A3 (2, 36.5) -> (0, 38.5) centre (0, 36.5) ccw
  line L10 (0, 38.5) -> (-38.5, 38.5)
  arc A4 (-38.5, 38.5) -> (-40.5, 36.5) centre (-38.5, 36.5) ccw
  line L11 (-40.5, 36.5) -> (-40.5, 15)
  line L12 (-38.8, 36.8) -> (-30.8, 36.8)
  line L13 (-30.8, 36.8) -> (-30.8, 34.4967)
  spline S1 degree 3 poles (-30.8, 34.4967) (-30.8, 34.2845) (-30.8711, 34.0401) (-31.1144, 33.5513) (-31.3774, 33.2489) (-31.6, 33) knots 0.417185 0.417185 0.417185 0.417185 0.480823 0.480823 0.581002 0.581002 0.581002 0.581002
  line L14 (-31.6, 33) -> (-38.8, 33)
  line L15 (-38.8, 33) -> (-38.8, 36.8)
  spline S2 degree 3 poles (-5.7, 33) (-5.9771, 33.2771) (-6.3039, 33.6152) (-6.6104, 34.1847) (-6.7, 34.4772) (-6.7, 34.7321) knots 0 0 0 0 0.117563 0.117563 0.194026 0.194026 0.194026 0.194026
  line L16 (-6.7, 34.7321) -> (-6.7, 36.8)
  line L17 (-6.7, 36.8) -> (0.3, 36.8)
  line L18 (0.3, 36.8) -> (0.3, 33)
  line L19 (0.3, 33) -> (-5.7, 33)
  circle A5 centre (-11, 25) radius 9.5
  circle A6 centre (-11, 25) radius 10
  line L20 (-6.7, 16.5289) -> (-6.7, 15.9717)
  line L21 (-4.0718, 18.5) -> (-3.4007, 18.5)
  dimension "d176" = 0.5
  constraint concentric A0 A5
  constraint coincident A0.end L3.end
  constraint coincident A6 L20.end
  constraint coincident L3 L20.end
  constraint coincident A0.start L0.start
  constraint coincident L0 L21.end
  constraint coincident A6 L21.end
extrude "Extrude30" cut sketch "Sketch28" along normal blind 7.8 contours L0 L3 A5 A6 L20 L21 bodies 2
sketch "Sketch29" plane through (0, 36.8, 0) normal (0, 1, 0) x (-1, 0, 0)
  line L0 (-6.7, -17.8) -> (0.3, -17.8)
  line L1 (0.3, -17.8) -> (0.3, -10)
  line L2 (0.3, -10) -> (-6.7, -10)
  line L3 (-6.7, -10) -> (-6.7, -17.8)
  circle A0 centre (-2.7, -14) radius 1.25
  dimension "d179" = 2.5
  dimension "d180" = 3
  dimension "d181" = 4
  measures "d179" diameter of A0
  measures "d180" distance of L1 A0.centre
  measures "d181" distance of L2 A0.centre
extrude "Extrude31" cut sketch "Sketch29" against normal blind 22.1 contours A0 bodies 2
move_body "Move6" bodies 2 to x (1, 0, 0) y (0, 1, 0) z (0, 0, 1) at (0, 0, -20)
sketch "Sketch30" plane through (0, 38.5, 0) normal (0, 1, 0) x (-1, 0, 0)
  line L0 (-38.5, -45.9) -> (0, -45.9)
  line L1 (0, -45.9) -> (0, -30)
  line L2 (0, -30) -> (-38.5, -30)
  line L3 (-38.5, -30) -> (-38.5, -45.9)
  circle A0 centre (-2.7, -34) radius 1.25
  circle A1 centre (-35, -34) radius 1.25
extrude "Extrude32" cut sketch "Sketch30" against normal blind 25.5 contours A0 | A1 bodies 3
sketch "Sketch31" plane through (0, 0, -30) normal (0, 0, -1) x (-1, 0, 0)
  line L0 (-3.4007, 18.5) -> (0.3, 18.5)
  line L1 (0.3, 18.5) -> (0.3, 14.7)
  line L2 (0.3, 14.7) -> (-6.7, 14.7)
  line L3 (-6.7, 14.7) -> (-6.7, 15.9717)
  arc A0 (-6.7, 15.9717) -> (-3.4007, 18.5) centre (-11, 25) ccw
  circle A1 centre (-11, 25) radius 9.5
  line L4 (-30.8, 14.7) -> (-38.8, 14.7)
  line L5 (-38.8, 14.7) -> (-38.8, 18.5)
  line L6 (-38.8, 18.5) -> (-31.6, 18.5)
  spline S0 degree 3 poles (-31.6, 18.5) (-31.3774, 18.2511) (-31.1144, 17.9487) (-30.8711, 17.4599) (-30.8, 17.2155) (-30.8, 17.0033) knots 0 0 0 0 0.100179 0.100179 0.163817 0.163817 0.163817 0.163817
  line L7 (-30.8, 17.0033) -> (-30.8, 14.7)
  arc A2 (-40.5, 15) -> (-38.5, 13) centre (-38.5, 15) ccw
  line L8 (-38.5, 13) -> (0, 13)
  arc A3 (0, 13) -> (2, 15) centre (0, 15) ccw
  line L9 (2, 15) -> (2, 36.5)
  arc A4 (2, 36.5) -> (0, 38.5) centre (0, 36.5) ccw
  line L10 (0, 38.5) -> (-38.5, 38.5)
  arc A5 (-38.5, 38.5) -> (-40.5, 36.5) centre (-38.5, 36.5) ccw
  line L11 (-40.5, 36.5) -> (-40.5, 15)
  line L12 (-38.8, 36.8) -> (-30.8, 36.8)
  line L13 (-30.8, 36.8) -> (-30.8, 34.4967)
  spline S1 degree 3 poles (-30.8, 34.4967) (-30.8, 34.2845) (-30.8711, 34.0401) (-31.1144, 33.5513) (-31.3774, 33.2489) (-31.6, 33) knots 0.417185 0.417185 0.417185 0.417185 0.480823 0.480823 0.581002 0.581002 0.581002 0.581002
  line L14 (-31.6, 33) -> (-38.8, 33)
  line L15 (-38.8, 33) -> (-38.8, 36.8)
  spline S2 degree 3 poles (-5.7, 33) (-5.9771, 33.2771) (-6.3039, 33.6152) (-6.6104, 34.1847) (-6.7, 34.4772) (-6.7, 34.7321) knots 0 0 0 0 0.117563 0.117563 0.194026 0.194026 0.194026 0.194026
  line L16 (-6.7, 34.7321) -> (-6.7, 36.8)
  line L17 (-6.7, 36.8) -> (0.3, 36.8)
  line L18 (0.3, 36.8) -> (0.3, 33)
  line L19 (0.3, 33) -> (-5.7, 33)
  line L20 (-30, 13.3) -> (0, 13.3)
  arc A6 (0, 13.3) -> (1.7, 15) centre (0, 15) ccw
  line L21 (1.7, 15) -> (1.7, 36.5)
  arc A7 (1.7, 36.5) -> (0, 38.2) centre (0, 36.5) ccw
  line L22 (0, 38.2) -> (-38.5, 38.2)
  arc A8 (-38.5, 38.2) -> (-40.2, 36.5) centre (-38.5, 36.5) ccw
  line L23 (-40.2, 36.5) -> (-40.2, 15)
  arc A9 (-40.2, 15) -> (-38.5, 13.3) centre (-38.5, 15) ccw
  line L24 (-38.5, 13.3) -> (-35, 13.3)
  line L25 (-35, 13.3) -> (-35, 17.5)
  arc A10 (-30, 17.5) -> (-35, 17.5) centre (-32.5, 17.5) ccw
  line L26 (-30, 17.5) -> (-30, 13.3)
  line L27 (-35, 13.3) -> (-35, 13)
  line L28 (-35, 13.3) -> (-38.5, 13.3)
  line L29 (-38.5, 13.3) -> (-38.5, 13)
  line L30 (-38.5, 13) -> (-35, 13)
  line L31 (-30, 13) -> (-30, 13.3)
  line L32 (-30, 13) -> (0, 13)
  line L33 (0, 13) -> (0, 13.3)
  line L34 (0, 13.3) -> (-30, 13.3)
  line L35 (-30, 13) -> (-30, 13.3)
  line L36 (-30, 13.3) -> (-30, 17.5)
  line L37 (-30, 17.5) -> (-30, 15)
  line L38 (-30, 15) -> (-30, 14.5)
  line L39 (-30, 14.5) -> (-30, 13)
  line L40 (-35, 14.5) -> (-35, 13)
  line L41 (-35, 13) -> (-35, 14.5)
  line L42 (-35, 14.5) -> (-30, 14.5)
  line L43 (-30, 14.5) -> (-30, 13)
  line L44 (-30, 13) -> (-35, 13)
  line L45 (-35, 13) -> (-35, 14.5)
  line L46 (-34.85, 14.5) -> (-34.85, 13)
  line L47 (-30.15, 14.5) -> (-30.15, 13)
  dimension "d186" = 0.15
  dimension "d187" = 0.15
  constraint horizontal L42
  constraint vertical L43
  constraint horizontal L44
  constraint vertical L45
  constraint coincident L31.start L32.start
  constraint coincident L40.start L41.end
  constraint vertical L46
  constraint coincident L42 L46.start
  constraint coincident L44 L46.end
  constraint coincident L42 L47.start
  constraint coincident L44 L47.end
  measures "d186" distance of L43 L47
  measures "d187" distance of L45 L46
extrude "Extrude33" add sketch "Sketch31" along normal blind 16.2 contours L8 L42 L44 L46 L47 bodies 2
sketch "Sketch32" plane through (0, 14.5, 0) normal (0, 1, 0) x (-1, 0, 0)
  line L0 (-30.15, -30) -> (-34.85, -30)
  line L1 (-34.85, -30) -> (-34.85, -46.2)
  line L2 (-34.85, -46.2) -> (-30.15, -46.2)
  line L3 (-30.15, -46.2) -> (-30.15, -30)
  circle A0 centre (-35, -34) radius 1.25
  line L4 (-38.8, -37.8) -> (-30.8, -37.8)
  line L5 (-30.8, -37.8) -> (-30.8, -30)
  line L6 (-30.8, -30) -> (-38.8, -30)
  line L7 (-38.8, -30) -> (-38.8, -37.8)
  line L8 (-34.8, -37.8) -> (-30.8, -37.8)
  line L9 (-30.8, -37.8) -> (-30.8, -30)
  line L10 (-30.8, -30) -> (-34.8, -30)
  line L11 (-34.8, -30) -> (-34.8, -37.8)
  constraint horizontal L8
  constraint vertical L9
  constraint horizontal L10
  constraint vertical L11
  constraint coincident L5.end L6.start
  constraint midpoint L4 L8.start
extrude "Extrude34" add sketch "Sketch32" along normal blind 0.2 contours L0 A0 L4 L5 L6 L8 L9 L10 L11 bodies 2
fillet "Fillet14" radius 0.5 2 edges at (32.8, 14.5, -37.8) (30.8, 14.5, -33.9) on bodies 2
sketch "Sketch33" plane through (0, 17.5, 0) normal (0, 1, 0) x (-1, 0, 0)
  circle A0 centre (-35, -34) radius 1.25
  line L0 (-31.6, -37.8) -> (-31.6, -31)
  line L1 (-31.6, -31) -> (-38.8, -31)
  line L2 (-38.8, -31) -> (-38.8, -37.8)
  line L3 (-38.8, -37.8) -> (-31.6, -37.8)
extrude "Extrude35" cut sketch "Sketch33" against normal blind 4.5 contours A0 bodies 2
fillet "Fillet15" radius 0.3 1 edges at (32.5, 13, -46.2) on bodies 2
move_body "Move7" bodies 2 to x (1, 0, 0) y (0, 1, 0) z (0, 0, 1) at (0, 0, 20)
move_face "OffsetFaces1" offset -0.2 1 faces at (12.8333, 38, -30) on bodies 3
fillet "Fillet16" radius 0.5 4 edges at (-0.3, 36.8, -13.9) (-0.3, 14.7, -13.9) (38.8, 36.8, -13.9) (38.8, 14.7, -13.95) on bodies 2
hidden bodies 1
equation "d68 = ( -42.5 / 2 ) * 1 mm"
equation "d96 = ( 8 / 2 ) * 1 mm + 0.2 mm"
named bodies: "Camera", "Lid", "Case", "Stand"
